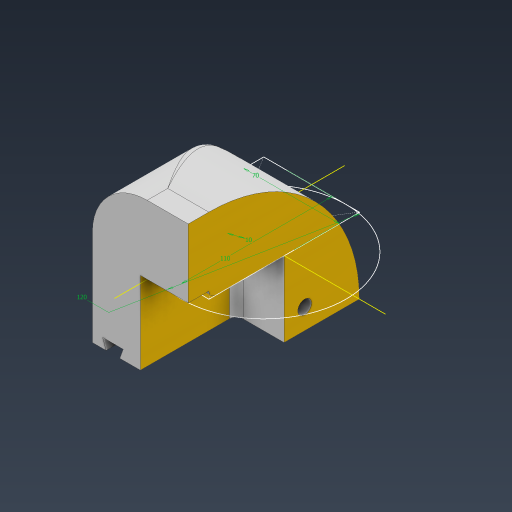
# Autodesk Inventor part: Уголок крышки
Saved by Autodesk Inventor 2023.2 (Build 272271030, 271C)
## iProperties
Created: 2025-04-26
Part Number: Уголок крышки
Material: Типовые
Document SubType Name: Modeling
Designer: Олег Коноваленко
Density: 1 g/cm^3
Appearance: По умолчанию
Author: Олег Коноваленко
Autodesk Inventor part; units mm, degrees
ref_plane "YZ Plane" through (0, 0, 0) normal (1, 0, 0) x (0, 1, 0)
ref_plane "XZ Plane" through (0, 0, 0) normal (0, 1, 0) x (-1, 0, 0)
ref_plane "XY Plane" through (0, 0, 0) normal (0, 0, 1) x (1, 0, 0)
sketch "Эскиз1" plane through (0, 0, 0) normal (0, 1, 0) x (-1, 0, 0)
  line L0 (35, -55) -> (35, 55)
  line L1 (35, 55) -> (-35, 55)
  line L2 (-35, 55) -> (-35, -55)
  line L3 (-35, -55) -> (35, -55)
  line L4 (-35, 55) -> (35, -55) construction
  line L5 (35, 55) -> (-35, -55) construction
  line L6 (-109, 0) -> (59, 0) projected
  line L7 (0, -79) -> (0, 89) projected
  circle A0 centre (-25, 5) radius 60
  circle A1 centre (-5, 5) radius 5
  point P0 (0, 0)
  point P1 (0, 0)
  point P2 (-35, 0)
  point P3 (0, 55)
  point P4 (-25, -55)
  point P5 (0, -55)
  point P6 (-35, -54.1608)
  point P7 (35, 0)
  point P8 (35, 5)
  point P9 (0, 0)
  point P10 (0, 5)
  point P11 (-5, 0)
  dimension "d1" = 70
  dimension "d2" = 110
  dimension "d20" = 120
  dimension "d40" = 10
  constraints: 12 end point, 4 tangent, 2 centre point, 2 midpoint, 2 perpendicular, 2 point on line, 1 vertical
  measures "d1" distance between parallel lines of L0 L2
  measures "d2" distance between parallel lines of L1 L3
  measures "d20" diameter of A0
  measures "d40" diameter of A1
extrude "Выдавливание1" add sketch "Эскиз1" along normal mid plane 110 contours A0 L1 L0 | A0 L6 L7 L1 | A0 L7 L6 | L7 A0 L2 L6 | L6 A1 L7 | L3 L2 A0
sketch "Эскиз4" plane through (35, -55, -55) normal (1, 0, 0) x (0, 0, -1)
  arc A0 (0, 0) -> (-110, 110) centre (-110, 0) ccw
  line L0 (-110, 110) -> (-60, 110) projected
  line L1 (-55, 110) -> (0, 110) projected
  line L2 (0, 0) -> (0, 110) projected
  line L3 (-60, 110) -> (-30, 110) projected
  line L4 (-110, 0) -> (-110, 110) projected
  point P0 (-55, 55)
  point P1 (0, 0.91)
  constraints: 2 point on circle, 1 centre point, 1 line through centre, 2 other
extrude "Выдавливание3" cut sketch "Эскиз4" against normal up to surface (70 mm away)
extrude "Выдавливание12" add sketch "Эскиз1" along normal up to surface contours L7 A1 L6 L2 L1 | A1 round surface about axis through (35, -55, 55) along (-1, 0, 0) radius 110 far side no
fillet "Сопряжение2" radius 5 1 edges at (17.5, 0, 55)
sketch "Эскиз7" plane through (-35, -55, 55) normal (0, 0, 1) x (1, 0, 0)
  line L0 (20, 0) -> (22.5, 7) projected
  line L1 (22.5, 7) -> (7.5, 7) projected
  line L2 (7.5, 7) -> (10, 0) projected
  line L3 (35, 0) -> (0, 0) projected
  point P0 (35, 55)
extrude "Выдавливание8" cut sketch "Эскиз7" against normal through all
sketch "Эскиз9" plane through (35, -55, 0) normal (1, 0, 0) x (0, 0, -1)
  circle A0 centre (15, 15) radius 5
  line L0 (55, 0) -> (0, 0) projected
  line L1 (0, 0) -> (0, 55) projected
  point P0 (0, 50)
  dimension "d52" = 10
  dimension "d53" = 15
  dimension "d54" = 15
  constraints: 1 centre point
  measures "d52" diameter of A0
  measures "d53" distance from line of L0 A0.centre
  measures "d54" distance from line of L1 A0.centre
extrude "Выдавливание10" cut sketch "Эскиз9" against normal blind 20
sketch "Эскиз13" plane through (-35, 55, 55) normal (0, 0, 1) x (1, 0, 0)
  line L0 (0, -110) -> (0, -12.0204) projected
  line L1 (0, -40) -> (40, -40)
  line L2 (40, -40) -> (40, 0)
  line L3 (0, 0) -> (70, 0) projected
  line L4 (0, 0) -> (0, -110) projected
  arc A0 (40, 0) -> (0, -40) centre (40, -40) ccw
  point P0 (35, -55)
  dimension "d66" = 40
  constraints: 4 end point, 3 perpendicular, 2 line through centre, 2 point on circle, 2 point on line, 1 centre point, 1 horizontal
  measures "d66" distance of L1.start L1.end
extrude "Выдавливание14" cut sketch "Эскиз13" against normal up to next contours L0 L4 L3 A0
sketch "Эскиз14" plane through (0, 5, 55) normal (0, 0, 1) x (1, 0, 0)
  arc A0 (5, 50) -> (-35, 10) centre (5, 10) ccw projected
  line L0 (-35, 10) -> (-35, -60) projected
  line L1 (-25, -60) -> (-35, -60) projected
  line L2 (-25, -60) -> (-27.5, -53) projected
  line L3 (-27.5, -53) -> (-12.5, -53) projected
  line L4 (-12.5, -53) -> (-15, -60) projected
  line L5 (0, -60) -> (-15, -60) projected
  line L6 (0, -60) -> (0, 0) projected
  line L7 (35, 0) -> (0, 0) projected
  line L8 (35, 0) -> (35, 50) projected
  line L9 (5, 50) -> (35, 50) projected
  point P0 (0, -5)
extrude "Выдавливание15" add sketch "Эскиз14" along normal blind 15
fillet "Сопряжение4" radius 5 4 edges at (-6.6486, -11.3626, -45.9741) (-34.227, 22.8257, -4.6001) (2.4976, 54.9216, 50.849) (-17.7829, 47.8776, 16.0617)
mirror "Зеркальное отражение2" [suppressed]
